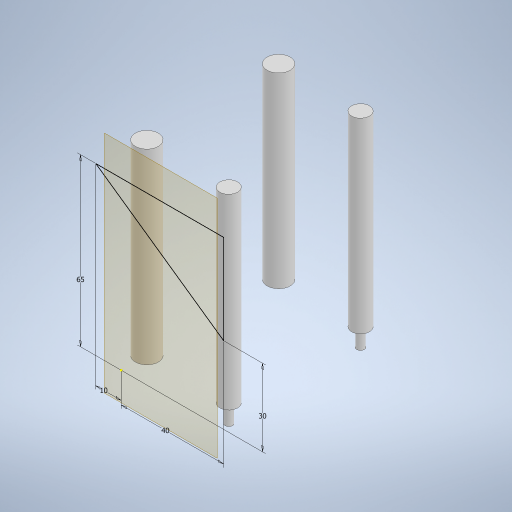
# Autodesk Inventor part: ControlPanel01
Saved by Autodesk Inventor 2024 (Build 280153000, 153)
## iProperties
Created: 2024-04-16
Part Number: ControlPanel01
Material: Generic
Document SubType Name: Modeling
Designer: ringl
Density: 1 g/cm^3
Appearance: Default
Author: ringl
Autodesk Inventor part; units mm, degrees
ref_plane "YZ Plane" through (0, 0, 0) normal (1, 0, 0) x (0, 1, 0)
ref_plane "XZ Plane" through (0, 0, 0) normal (0, 1, 0) x (-1, 0, 0)
sketch "Sketch1" plane through (0, 0, 0) normal (0, 1, 0) x (-1, 0, 0)
  circle A0 centre (0, 0) radius 4.5
  circle A1 centre (0, 0) radius 3.25
  circle A2 centre (0, -51.5) radius 3.25
  circle A3 centre (0, -51.5) radius 4.5
  circle A4 centre (-32, 0) radius 3.5
  circle A5 centre (-32, -51.5) radius 3.5
  dimension "d0" = 9
  dimension "d1" = 6.5
  dimension "d2" = 6.5
  dimension "d3" = 9
  dimension "d4" = 7
  dimension "d5" = 7
  dimension "d6" = 51.5
  dimension "d7" = 32
  constraints: 6 centre point, 3 coincident, 2 horizontal alignment, 2 vertical alignment
  measures "d0" diameter of A0
  measures "d1" diameter of A1
  measures "d2" diameter of A2
  measures "d3" diameter of A3
  measures "d4" diameter of A4
  measures "d5" diameter of A5
  measures "d6" distance of A2.centre point (0, 0)
  measures "d7" distance of A5.centre A2.centre
extrude "Extrusion1" add sketch "Sketch1" along normal blind 6
sketch "Sketch2" plane through (32, 0, 0) normal (0, -1, 0) x (1, 0, 0)
  circle A0 centre (0, 0) radius 1.5
  circle A1 centre (0, -51.5) radius 3.5 projected
  circle A2 centre (0, -51.5) radius 1.5
  point P0 (-32, 0)
  dimension "d10" = 3
  dimension "d11" = 3
  constraints: 2 centre point, 1 coincident
  measures "d10" diameter of A0
  measures "d11" diameter of A2
extrude "Extrusion2" add sketch "Sketch2" along normal blind 7 contours A0 | A2
sketch "Sketch3" plane through (0, 6, 0) normal (0, 1, 0) x (1, 0, 0)
  point P0 (0, 0)
sketch "Sketch4" plane through (0, 6, 0) normal (0, 1, 0) x (1, 0, 0)
  circle A0 centre (0, 0) radius 3.25 projected
  circle A1 centre (0, 0) radius 3.25
  circle A2 centre (0, 0) radius 4.5
  circle A3 centre (0, 51.5) radius 3.25 projected
  circle A4 centre (0, 51.5) radius 3.25
  circle A5 centre (0, 51.5) radius 4.5
  circle A6 centre (32, 0) radius 3.5 projected
  circle A7 centre (32, 51.5) radius 3.5 projected
  circle A8 centre (32, 0) radius 3.5
  circle A9 centre (32, 51.5) radius 1.5 projected
  circle A10 centre (32, 51.5) radius 3.5
  constraints: 6 centre point, 6 coincident, 3 concentric
extrude "Extrusion3" add sketch "Sketch4" along normal blind 7 contours A2 | A5 | A6 | A7 | A9
sketch "Sketch5" plane through (0, 13, 0) normal (0, 1, 0) x (1, 0, 0)
  circle A0 centre (32, 0) radius 1.5 projected
  circle A1 centre (32, 0) radius 3.5
  circle A2 centre (0, 0) radius 4.5
  circle A3 centre (0, 51.5) radius 3.25 projected
  circle A4 centre (0, 51.5) radius 4.5
  circle A5 centre (32, 51.5) radius 1.5 projected
  circle A6 centre (32, 51.5) radius 3.5
  dimension "d18" = 7
  dimension "d19" = 7
  dimension "d20" = 9
  dimension "d21" = 9
  constraints: 4 centre point, 4 coincident
  measures "d18" diameter of A1
  measures "d19" diameter of A6
  measures "d20" diameter of A4
  measures "d21" diameter of A2
extrude "Extrusion4" add sketch "Sketch5" along normal blind 60 contours A0 | A1 | A2 | A3 | A4 | A5 | A6
ref_plane "Work Plane1" through (0, 0, 10) normal (0, 0, 1) x (1, 0, 0)
sketch "Sketch7" plane through (0, 0, 10) normal (0, 0, 1) x (1, 0, 0)
  point P0 (0, 0)
sketch "Sketch8" plane through (0, 0, 10) normal (0, 0, 1) x (1, 0, 0)
  line L0 (40, 30) -> (-10, 65)
  line L1 (-10, 65) -> (40, 65)
  line L2 (40, 65) -> (40, 30)
  point P0 (0, 0)
  dimension "d23" = 30
  dimension "d24" = 65
  dimension "d25" = 10
  dimension "d26" = 40
  constraints: 6 end point, 1 horizontal, 1 perpendicular
  measures "d23" vertical distance of point (0, 0) L0.start
  measures "d24" vertical distance of point (0, 0) L0.end
  measures "d25" horizontal distance of point (0, 0) L0.end
  measures "d26" horizontal distance of point (0, 0) L0.start
body "Solid1"
